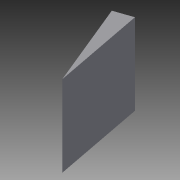
# Autodesk Inventor part: Ramp base
Saved by Autodesk Inventor 2014 (Build 180170000, 170)
## iProperties
Created: 2014-01-31
Part Number: Ramp base
Material: Generic
Document SubType Name: Modeling
Designer: JosephLyons
Density: 1 g/cm^3
Appearance: Default
Author: JosephLyons
Autodesk Inventor part; units mm, degrees
ref_plane "YZ Plane" through (0, 0, 0) normal (1, 0, 0) x (0, 1, 0)
ref_plane "XZ Plane" through (0, 0, 0) normal (0, 1, 0) x (-1, 0, 0)
ref_plane "XY Plane" through (0, 0, 0) normal (0, 0, 1) x (1, 0, 0)
sketch "Sketch1" plane through (0, 0, 0) normal (0, 1, 0) x (-1, 0, 0)
  line L0 (-975.868, 547.4737) -> (-799.1025, -369.9743)
  line L1 (-799.1025, -369.9743) -> (-623.3345, -309.7763)
  line L2 (-623.3345, -309.7763) -> (-975.868, 547.4737)
  point P0 (0, 0)
  dimension "d2" = 82
  dimension "d3" = 917.448
  dimension "d4" = 175.768
  dimension "d5" = 857.25
  constraints: 6 end point
  measures "d2" angle of L1 L0
  measures "d3" vertical distance of L0.start L0.end
  measures "d4" horizontal distance of L0.end L1.end
  measures "d5" vertical distance of L1.end L0.start
extrude "Extrusion1" add sketch "Sketch1" along normal blind 825.5
body "Solid1"
